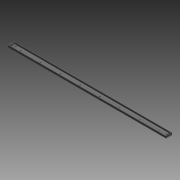
# Autodesk Inventor part: FBW2560R+640 L Rail
Saved by Autodesk Inventor 2011 SP1 (Build 150282100, 282)
## iProperties
Created: 2018-02-17
Part Number: FBW2560R+640 L Rail
Catalog Web Link: www.cadenas.de
Description: FBW2560RR-Satinless Steel Compact Type FBW2560XR
Vendor: THK
Document SubType Name: Modeling
Designer: psAdmin
Manufacturer: THK
Mass: 38.8329 g
Surface Area: 529.867 cm^2
Volume: 38.8329 cm^3
Density: 1 g/cm^3
Category: PARTsolutions
Company: THK
Title: FBW2560R+640 L Rail
Author: Cadenas PARTsolutions
Comments: Satinless Steel Compact Type FBW2560XR
PSOL_IDENT_0: {$CADENAS_DATA\23d-libs\thk\linear_motion_systems\slide_pack\perpetual_lm_type_fbw\stainless_steel_c
PSOL_IDENT_1: ompact_type_fbw2560r\fbw_2560r_rail.prj},183 {VTYP=3D},{NB=FBW2560R+640 L Rail},{LINA=FBW2560R+640 L
PSOL_IDENT_2: Rail},{NN=FBW2560RR},{DATE=22.12.2017 01:25:51},{GEOMDATE=04.07.2007 12:12:00},{VERSION=},{LINEID=7
PSOL_IDENT_3: 0},{LINESUBID=-1},{WBVAR=}  {NB=FBW2560R+640 L Rail},{LINA=FBW2560R+640 L Rail},{KT=DUMMY},{IDNR=},{
PSOL_IDENT_4: L=640},{N1=7},{G=40},{WOS=568},{WS=563},{M=290}
NN: FBW2560RR
NT: Satinless Steel Compact Type FBW2560XR
NB: FBW2560R+640 L Rail
NBSYN: FBW2560R+$L. L Rail
LINA: FBW2560R+640 L Rail
L: 640
N1: 7
G: 40
WOS: 568
WS: 563
M: 290
SUPPLIER: THK
ARTICLENO: FBW2560R+640 L Rail
BOMINFO: FBW2560R+640 L Rail
CREATOR: CADENAS GmbH
Autodesk Inventor part; units mm, degrees
sketch "Sketch_1" plane through (0, 0, 0) normal (1, 0, 0) x (0, 1, 0)
  line L0 (10.9, 9.22) -> (10.9, 2.5)
  arc A0 (9.9, 1.5) -> (10.9, 2.5) centre (9.9, 2.5) ccw
  line L1 (9.9, 1.5) -> (-9.9, 1.5)
  arc A1 (-10.9, 2.5) -> (-9.9, 1.5) centre (-9.9, 2.5) ccw
  line L2 (-10.9, 2.5) -> (-10.9, 9.22)
  line L3 (-10.9, 9.22) -> (-12.4, 9.22)
  line L4 (-12.4, 9.22) -> (-12.4, 2)
  arc A2 (-12.4, 2) -> (-10.4, 0) centre (-10.4, 2) ccw
  line L5 (-10.4, 0) -> (10.4, 0)
  arc A3 (10.4, 0) -> (12.4, 2) centre (10.4, 2) ccw
  line L6 (12.4, 2) -> (12.4, 9.22)
  line L7 (12.4, 9.22) -> (10.9, 9.22)
  constraints: 16 end point, 8 point on circle, 4 centre point
extrude "Extrusion1" add sketch "Sketch_1" along normal blind 640
sketch "Sketch_5" plane through (0, 0, 1.5) normal (0, 0, 1) x (1, 0, 0)
  arc A0 (4.5, -8) -> (6.5, -10) centre (6.5, -8) ccw
  line L0 (6.5, -10) -> (11.5, -10)
  arc A1 (11.5, -10) -> (13.5, -8) centre (11.5, -8) ccw
  line L1 (13.5, -8) -> (13.5, 8)
  arc A2 (13.5, 8) -> (11.5, 10) centre (11.5, 8) ccw
  line L2 (11.5, 10) -> (6.5, 10)
  arc A3 (6.5, 10) -> (4.5, 8) centre (6.5, 8) ccw
  line L3 (4.5, 8) -> (4.5, -8)
  constraints: 8 end point, 8 point on circle, 4 centre point
extrude "Extrusion2" add sketch "Sketch_5" along normal blind 2
sketch "Sketch_8" plane through (9, 0, 0) normal (1, 0, 0) x (0, 0, -1)
  line L0 (-3.45, 6.85) -> (-3.45, 5.15)
  line L1 (-3.45, 5.15) -> (-1.6, 5.7)
  line L2 (-1.6, 5.7) -> (-1.6, 6.3)
  line L3 (-1.6, 6.3) -> (-3.45, 6.85)
  constraints: 8 end point
extrude "Extrusion3" cut sketch "Sketch_8" along normal mid plane 0.4
sketch "Sketch_9" plane through (0, 6, 0) normal (0, 1, 0) x (1, 0, 0)
  line L0 (8.15, -3.45) -> (9.85, -3.45)
  line L1 (9.85, -3.45) -> (9.3, -1.6)
  line L2 (9.3, -1.6) -> (8.7, -1.6)
  line L3 (8.7, -1.6) -> (8.15, -3.45)
  constraints: 8 end point
extrude "Extrusion4" cut sketch "Sketch_9" along normal mid plane 0.4
sketch "Sketch_10" plane through (9, 0, 0) normal (1, 0, 0) x (0, 0, -1)
  line L0 (-3.45, -5.15) -> (-3.45, -6.85)
  line L1 (-3.45, -6.85) -> (-1.6, -6.3)
  line L2 (-1.6, -6.3) -> (-1.6, -5.7)
  line L3 (-1.6, -5.7) -> (-3.45, -5.15)
  constraints: 8 end point
extrude "Extrusion5" cut sketch "Sketch_10" along normal mid plane 0.4
sketch "Sketch_11" plane through (0, -6, 0) normal (0, 1, 0) x (1, 0, 0)
  line L0 (8.15, -3.45) -> (9.85, -3.45)
  line L1 (9.85, -3.45) -> (9.3, -1.6)
  line L2 (9.3, -1.6) -> (8.7, -1.6)
  line L3 (8.7, -1.6) -> (8.15, -3.45)
  constraints: 8 end point
extrude "Extrusion6" cut sketch "Sketch_11" along normal mid plane 0.4
sketch "Sketch_12" plane through (0, 0, 3.5) normal (0, 0, 1) x (1, 0, 0)
  arc A0 (0.4, -7.5) -> (2.4, -9.5) centre (2.4, -7.5) ccw
  line L0 (2.4, -9.5) -> (4, -9.5)
  arc A1 (4, -9.5) -> (6, -7.5) centre (4, -7.5) ccw
  line L1 (6, -7.5) -> (6, 7.5)
  arc A2 (6, 7.5) -> (4, 9.5) centre (4, 7.5) ccw
  line L2 (4, 9.5) -> (2.4, 9.5)
  arc A3 (2.4, 9.5) -> (0.4, 7.5) centre (2.4, 7.5) ccw
  line L3 (0.4, 7.5) -> (0.4, -7.5)
  line L4 (1.9, 8) -> (1.9, -8)
  line L5 (1.9, -8) -> (4.5, -8)
  line L6 (4.5, -8) -> (4.5, 8)
  line L7 (4.5, 8) -> (1.9, 8)
  constraints: 16 end point, 8 point on circle, 4 centre point
extrude "Extrusion7" add sketch "Sketch_12" along normal blind 5
sketch "Sketch_13" plane through (0, 0, 1.5) normal (0, 0, 1) x (1, 0, 0)
  line L0 (626.5, 8) -> (626.5, -8)
  arc A0 (626.5, -8) -> (628.5, -10) centre (628.5, -8) ccw
  line L1 (628.5, -10) -> (633.5, -10)
  arc A1 (633.5, -10) -> (635.5, -8) centre (633.5, -8) ccw
  line L2 (635.5, -8) -> (635.5, 8)
  arc A2 (635.5, 8) -> (633.5, 10) centre (633.5, 8) ccw
  line L3 (633.5, 10) -> (628.5, 10)
  arc A3 (628.5, 10) -> (626.5, 8) centre (628.5, 8) ccw
  constraints: 8 end point, 8 point on circle, 4 centre point
extrude "Extrusion8" add sketch "Sketch_13" along normal blind 2
sketch "Sketch_16" plane through (631, 0, 0) normal (1, 0, 0) x (0, 0, -1)
  line L0 (-3.45, 6.85) -> (-3.45, 5.15)
  line L1 (-3.45, 5.15) -> (-1.6, 5.7)
  line L2 (-1.6, 5.7) -> (-1.6, 6.3)
  line L3 (-1.6, 6.3) -> (-3.45, 6.85)
  constraints: 8 end point
extrude "Extrusion9" cut sketch "Sketch_16" along normal mid plane 0.4
sketch "Sketch_17" plane through (0, 6, 0) normal (0, 1, 0) x (1, 0, 0)
  line L0 (630.15, -3.45) -> (631.85, -3.45)
  line L1 (631.85, -3.45) -> (631.3, -1.6)
  line L2 (631.3, -1.6) -> (630.7, -1.6)
  line L3 (630.7, -1.6) -> (630.15, -3.45)
  constraints: 8 end point
extrude "Extrusion10" cut sketch "Sketch_17" along normal mid plane 0.4
sketch "Sketch_18" plane through (631, 0, 0) normal (1, 0, 0) x (0, 0, -1)
  line L0 (-3.45, -5.15) -> (-3.45, -6.85)
  line L1 (-3.45, -6.85) -> (-1.6, -6.3)
  line L2 (-1.6, -6.3) -> (-1.6, -5.7)
  line L3 (-1.6, -5.7) -> (-3.45, -5.15)
  constraints: 8 end point
extrude "Extrusion11" cut sketch "Sketch_18" along normal mid plane 0.4
sketch "Sketch_19" plane through (0, -6, 0) normal (0, 1, 0) x (1, 0, 0)
  line L0 (630.15, -3.45) -> (631.85, -3.45)
  line L1 (631.85, -3.45) -> (631.3, -1.6)
  line L2 (631.3, -1.6) -> (630.7, -1.6)
  line L3 (630.7, -1.6) -> (630.15, -3.45)
  constraints: 8 end point
extrude "Extrusion12" cut sketch "Sketch_19" along normal mid plane 0.4
sketch "Sketch_20" plane through (0, 0, 3.5) normal (0, 0, 1) x (1, 0, 0)
  line L0 (634, 7.5) -> (634, -7.5)
  arc A0 (634, -7.5) -> (636, -9.5) centre (636, -7.5) ccw
  line L1 (636, -9.5) -> (637.6, -9.5)
  arc A1 (637.6, -9.5) -> (639.6, -7.5) centre (637.6, -7.5) ccw
  line L2 (639.6, -7.5) -> (639.6, 7.5)
  arc A2 (639.6, 7.5) -> (637.6, 9.5) centre (637.6, 7.5) ccw
  line L3 (637.6, 9.5) -> (636, 9.5)
  arc A3 (636, 9.5) -> (634, 7.5) centre (636, 7.5) ccw
  line L4 (635.5, -8) -> (638.1, -8)
  line L5 (638.1, -8) -> (638.1, 8)
  line L6 (638.1, 8) -> (635.5, 8)
  line L7 (635.5, 8) -> (635.5, -8)
  constraints: 16 end point, 8 point on circle, 4 centre point
extrude "Extrusion13" add sketch "Sketch_20" along normal blind 5
sketch "Sketch_4_ALT_Drilling_1" plane through (9, 0, 0) normal (1, 0, 0) x (0, 0, -1)
  line L0 (-3.45, 6) -> (-3.5, 6)
  line L1 (-3.5, 6) -> (-3.5, 7.5)
  line L2 (-3.5, 7.5) -> (-3.45, 7.5)
  line L3 (-3.45, 7.5) -> (-3.45, 6)
  line L4 (-3.45, 6) -> (-3.5, 6)
  constraints: 10 end point
revolve "Revolution1" cut sketch "Sketch_4_ALT_Drilling_1" angle 360 about axis through (9, 6, 3.45) along (0, 0, -1)
sketch "Sketch_6_ALT_Drilling_2" plane through (9, 0, 0) normal (1, 0, 0) x (0, 0, -1)
  line L0 (-3.45, -6) -> (-3.5, -6)
  line L1 (-3.5, -6) -> (-3.5, -4.5)
  line L2 (-3.5, -4.5) -> (-3.45, -4.5)
  line L3 (-3.45, -4.5) -> (-3.45, -6)
  line L4 (-3.45, -6) -> (-3.5, -6)
  constraints: 10 end point
revolve "Revolution2" cut sketch "Sketch_6_ALT_Drilling_2" angle 360 about axis through (9, -6, 3.45) along (0, 0, -1)
sketch "Sketch_7_ALT_Drilling_3" plane through (631, 0, 0) normal (1, 0, 0) x (0, 0, -1)
  line L0 (-3.45, 6) -> (-3.5, 6)
  line L1 (-3.5, 6) -> (-3.5, 7.5)
  line L2 (-3.5, 7.5) -> (-3.45, 7.5)
  line L3 (-3.45, 7.5) -> (-3.45, 6)
  line L4 (-3.45, 6) -> (-3.5, 6)
  constraints: 10 end point
revolve "Revolution3" cut sketch "Sketch_7_ALT_Drilling_3" angle 360 about axis through (631, 6, 3.45) along (0, 0, -1)
sketch "Sketch_14_ALT_Drilling_4" plane through (631, 0, 0) normal (1, 0, 0) x (0, 0, -1)
  line L0 (-3.45, -6) -> (-3.5, -6)
  line L1 (-3.5, -6) -> (-3.5, -4.5)
  line L2 (-3.5, -4.5) -> (-3.45, -4.5)
  line L3 (-3.45, -4.5) -> (-3.45, -6)
  line L4 (-3.45, -6) -> (-3.5, -6)
  constraints: 10 end point
revolve "Revolution4" cut sketch "Sketch_14_ALT_Drilling_4" angle 360 about axis through (631, -6, 3.45) along (0, 0, -1)
sketch "Sketch_15_ALT_Drilling_5" plane through (17, 0, 0) normal (1, 0, 0) x (0, 0, -1)
  line L0 (0, 6) -> (-1.5, 6)
  line L1 (-1.5, 6) -> (-1.5, 7.6)
  line L2 (-1.5, 7.6) -> (0, 7.6)
  line L3 (0, 7.6) -> (0, 6)
  line L4 (0, 6) -> (-1.5, 6)
  constraints: 10 end point
revolve "Revolution5" cut sketch "Sketch_15_ALT_Drilling_5" angle 360 about axis through (17, 6, 0) along (0, 0, -1)
sketch "Sketch_22_ALT_Drilling_6" plane through (17, 0, 0) normal (1, 0, 0) x (0, 0, -1)
  line L0 (0, -6) -> (-1.5, -6)
  line L1 (-1.5, -6) -> (-1.5, -4.4)
  line L2 (-1.5, -4.4) -> (0, -4.4)
  line L3 (0, -4.4) -> (0, -6)
  line L4 (0, -6) -> (-1.5, -6)
  constraints: 10 end point
revolve "Revolution6" cut sketch "Sketch_22_ALT_Drilling_6" angle 360 about axis through (17, -6, 0) along (0, 0, -1)
sketch "Sketch_23_ALT_Drilling_7" plane through (623, 0, 0) normal (1, 0, 0) x (0, 0, -1)
  line L0 (0, 6) -> (-1.5, 6)
  line L1 (-1.5, 6) -> (-1.5, 7.6)
  line L2 (-1.5, 7.6) -> (0, 7.6)
  line L3 (0, 7.6) -> (0, 6)
  line L4 (0, 6) -> (-1.5, 6)
  constraints: 10 end point
revolve "Revolution7" cut sketch "Sketch_23_ALT_Drilling_7" angle 360 about axis through (623, 6, 0) along (0, 0, -1)
sketch "Sketch_24_ALT_Drilling_8" plane through (623, 0, 0) normal (1, 0, 0) x (0, 0, -1)
  line L0 (0, -6) -> (-1.5, -6)
  line L1 (-1.5, -6) -> (-1.5, -4.4)
  line L2 (-1.5, -4.4) -> (0, -4.4)
  line L3 (0, -4.4) -> (0, -6)
  line L4 (0, -6) -> (-1.5, -6)
  constraints: 10 end point
revolve "Revolution8" cut sketch "Sketch_24_ALT_Drilling_8" angle 360 about axis through (623, -6, 0) along (0, 0, -1)
sketch "Sketch_2" plane through (0, 0, 1.5) normal (0, 0, 1) x (1, 0, 0)
  arc A0 (39.65, 2.3) -> (39.65, -2.3) centre (39.65, 0) ccw
  line L0 (39.65, -2.3) -> (40.35, -2.3)
  arc A1 (40.35, -2.3) -> (40.35, 2.3) centre (40.35, 0) ccw
  line L1 (40.35, 2.3) -> (39.65, 2.3)
  constraints: 4 end point, 4 point on circle, 2 centre point
extrude "Extrusion14" cut sketch "Sketch_2" against normal blind 2.3
sketch "Pattern_1_SKETCH_1" plane through (0, 0, 1.5) normal (0, 0, 1) x (1, 0, 0)
  arc A0 (119.65, 2.3) -> (119.65, -2.3) centre (119.65, 0) ccw
  line L0 (119.65, -2.3) -> (120.35, -2.3)
  arc A1 (120.35, -2.3) -> (120.35, 2.3) centre (120.35, 0) ccw
  line L1 (120.35, 2.3) -> (119.65, 2.3)
  constraints: 4 end point, 4 point on circle, 2 centre point
sketch "Pattern_1_SKETCH_2" plane through (0, 0, 1.5) normal (0, 0, 1) x (1, 0, 0)
  arc A0 (199.65, 2.3) -> (199.65, -2.3) centre (199.65, 0) ccw
  line L0 (199.65, -2.3) -> (200.35, -2.3)
  arc A1 (200.35, -2.3) -> (200.35, 2.3) centre (200.35, 0) ccw
  line L1 (200.35, 2.3) -> (199.65, 2.3)
  constraints: 4 end point, 4 point on circle, 2 centre point
sketch "Pattern_1_SKETCH_3" plane through (0, 0, 1.5) normal (0, 0, 1) x (1, 0, 0)
  arc A0 (279.65, 2.3) -> (279.65, -2.3) centre (279.65, 0) ccw
  line L0 (279.65, -2.3) -> (280.35, -2.3)
  arc A1 (280.35, -2.3) -> (280.35, 2.3) centre (280.35, 0) ccw
  line L1 (280.35, 2.3) -> (279.65, 2.3)
  constraints: 4 end point, 4 point on circle, 2 centre point
sketch "Pattern_1_SKETCH_4" plane through (0, 0, 1.5) normal (0, 0, 1) x (1, 0, 0)
  arc A0 (359.65, 2.3) -> (359.65, -2.3) centre (359.65, 0) ccw
  line L0 (359.65, -2.3) -> (360.35, -2.3)
  arc A1 (360.35, -2.3) -> (360.35, 2.3) centre (360.35, 0) ccw
  line L1 (360.35, 2.3) -> (359.65, 2.3)
  constraints: 4 end point, 4 point on circle, 2 centre point
sketch "Pattern_1_SKETCH_5" plane through (0, 0, 1.5) normal (0, 0, 1) x (1, 0, 0)
  arc A0 (439.65, 2.3) -> (439.65, -2.3) centre (439.65, 0) ccw
  line L0 (439.65, -2.3) -> (440.35, -2.3)
  arc A1 (440.35, -2.3) -> (440.35, 2.3) centre (440.35, 0) ccw
  line L1 (440.35, 2.3) -> (439.65, 2.3)
  constraints: 4 end point, 4 point on circle, 2 centre point
sketch "Pattern_1_SKETCH_6" plane through (0, 0, 1.5) normal (0, 0, 1) x (1, 0, 0)
  arc A0 (519.65, 2.3) -> (519.65, -2.3) centre (519.65, 0) ccw
  line L0 (519.65, -2.3) -> (520.35, -2.3)
  arc A1 (520.35, -2.3) -> (520.35, 2.3) centre (520.35, 0) ccw
  line L1 (520.35, 2.3) -> (519.65, 2.3)
  constraints: 4 end point, 4 point on circle, 2 centre point
sketch "Pattern_1_SKETCH_7" plane through (0, 0, 1.5) normal (0, 0, 1) x (1, 0, 0)
  arc A0 (599.65, 2.3) -> (599.65, -2.3) centre (599.65, 0) ccw
  line L0 (599.65, -2.3) -> (600.35, -2.3)
  arc A1 (600.35, -2.3) -> (600.35, 2.3) centre (600.35, 0) ccw
  line L1 (600.35, 2.3) -> (599.65, 2.3)
  constraints: 4 end point, 4 point on circle, 2 centre point
extrude "Extrusion15" cut sketch "Pattern_1_SKETCH_1" against normal blind 2.3
extrude "Extrusion16" cut sketch "Pattern_1_SKETCH_2" against normal blind 2.3
extrude "Extrusion17" cut sketch "Pattern_1_SKETCH_3" against normal blind 2.3
extrude "Extrusion18" cut sketch "Pattern_1_SKETCH_4" against normal blind 2.3
extrude "Extrusion19" cut sketch "Pattern_1_SKETCH_5" against normal blind 2.3
extrude "Extrusion20" cut sketch "Pattern_1_SKETCH_6" against normal blind 2.3
extrude "Extrusion21" cut sketch "Pattern_1_SKETCH_7" against normal blind 2.3
ref_plane "rail_ip1_XY" through (3, 0, 0) normal (1, 0, 0) x (0, 0, -1)
ref_plane "rail_ip1_YZ" through (3, 0, 0) normal (0, 0, -1) x (0, 1, 0)
ref_plane "rail_ip1_ZX" through (3, 0, 0) normal (0, 1, 0) x (1, 0, 0)
body "Solid1"
